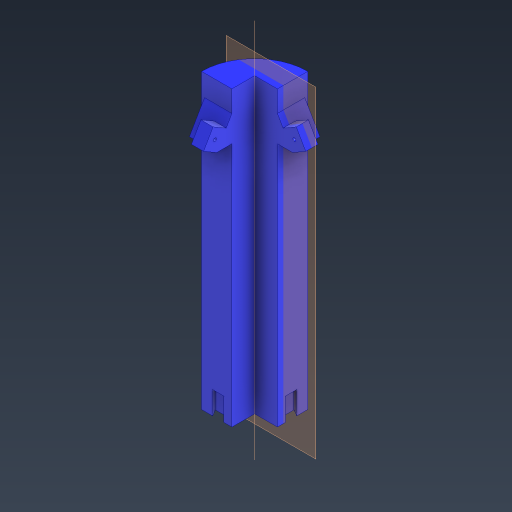
# Autodesk Inventor part: Край стен
Saved by Autodesk Inventor 2023.2 (Build 272271030, 271C)
## iProperties
Created: 2025-08-19
Part Number: Край стен
Material: Типовые
Document SubType Name: Modeling
Designer: Олег Коноваленко
Density: 1 g/cm^3
Appearance: Синий — малярная краска — глянцевая
Mass: 1127.71 g
Surface Area: 1041.8 cm^2
Volume: 1127.71 cm^3
Author: Олег Коноваленко
Autodesk Inventor part; units mm, degrees
ref_plane "YZ Plane" through (0, 0, 0) normal (1, 0, 0) x (0, 1, 0)
ref_plane "XZ Plane" through (0, 0, 0) normal (0, 1, 0) x (-1, 0, 0)
ref_plane "XY Plane" through (0, 0, 0) normal (0, 0, 1) x (1, 0, 0)
sketch "Эскиз1" plane through (0, 0, 0) normal (0, 1, 0) x (-1, 0, 0)
  line L0 (-39.7487, 9.7487) -> (-39.7487, -30.2513)
  line L1 (-9.7487, 9.7487) -> (-39.7487, 9.7487)
  line L2 (-9.7487, 9.7487) -> (-9.7487, 39.7487)
  line L3 (-9.7487, 39.7487) -> (30.2513, 39.7487)
  arc A0 (-39.7487, -30.2513) -> (30.2513, 39.7487) centre (-39.7487, 39.7487) ccw
  line L4 (-9.7487, 9.7487) -> (9.7487, -9.7487) construction
  point P0 (0, 0)
  point P1 (0, 0)
  dimension "d27" = 40
  dimension "d83" = 30
  constraints: 10 end point, 4 perpendicular, 3 point on circle, 2 line through centre, 1 centre point, 1 coincident, 1 horizontal, 1 midpoint, 1 vertical
  measures "d27" distance of L0.start L0.end
  measures "d83" distance of L1.start L0.start
extrude "Выдавливание16" add sketch "Эскиз1" along normal mid plane 386
ref_plane "РабПлоскость13" through (39.7487, 193, 39.7487) normal (-0.7071068, 0, 0.7071068) x (0, -1, 0)
sketch "Эскиз34" plane through (39.7487, 193, 39.7487) normal (-0.7071068, 0, 0.7071068) x (0, -1, 0)
  line L0 (-30, -100) -> (416, -100)
  line L1 (416, -100) -> (416, 8.7868)
  line L2 (416, 8.7868) -> (-30, 8.7868)
  line L3 (-30, 8.7868) -> (-30, -100)
  line L4 (386, -70) -> (0, -70) projected
  line L5 (386, -21.2132) -> (0, -21.2132) projected
  line L6 (386, -21.2132) -> (386, -49.4975) projected
  line L7 (0, -49.4975) -> (0, -21.2132) projected
  point P0 (193, -56.2132)
  dimension "d102" = 30
  dimension "d103" = 30
  dimension "d104" = 30
  dimension "d105" = 30
  constraints: 8 end point, 2 parallel, 1 horizontal, 1 perpendicular
  measures "d102" distance between parallel lines of L3 L7
  measures "d103" distance between parallel lines of L4 L0
  measures "d104" distance between parallel lines of L5 L2
  measures "d105" distance between parallel lines of L1 L6
sketch "Эскиз36" plane through (0, -193, 0) normal (0, -1, 0) x (1, 0, 0)
  line L0 (39.7487, 9.7487) -> (39.7487, -30.2513)
  line L1 (31.0885, -20.7513) -> (39.7487, -15.7513)
  line L2 (31.0885, 4.2487) -> (31.0885, -20.7513)
  line L3 (39.7487, -0.7513) -> (31.0885, 4.2487)
  point P0 (0, 0)
  constraints: 8 end point, 2 vertical, 8 other
extrude "Выдавливание25" cut sketch "Эскиз36" against normal blind 30
extrude "Выдавливание23" [suppressed]
mirror "Зеркальное отражение4" about plane through (39.7487, 193, 39.7487) normal (-0.7071068, 0, 0.7071068) of "Выдавливание25"
sketch "Эскиз37" plane through (9.7487, -193, 39.7487) normal (1, 0, 0) x (0, 0, -1)
  line L0 (-8.2128, 343.7788) -> (-180.7128, 45)
  line L1 (0, 0) -> (0, 386) projected
  line L2 (0, 358.0038) -> (-20, 323.3628)
  line L3 (-20, 323.3628) -> (0, 323.3628)
  point P0 (39.7487, 193)
  point P1 (-20, 323.3628)
  dimension "d112" = 30
  dimension "d113" = 20
  constraints: 6 end point, 3 point on line, 1 horizontal, 3 other
  measures "d112" angle of L1 L2
  measures "d113" distance of L2.end L3.end
ref_plane "РабПлоскость14" through (-26.2513, -147.25, 49.2606) normal (-1, 0, 0) x (0, 0.5, 0.8660254)
extrude "Выдавливание26" add sketch "Эскиз37" against normal up to surface (36 mm away)
sketch "Эскиз38" plane through (-26.2513, 130.3628, 59.7487) normal (0, 0.5, 0.8660254) x (1, 0, 0)
  line L0 (36, 0) -> (36, 10) projected
  line L1 (36, 0) -> (20, 0)
  line L2 (20, 0) -> (20, 25)
  line L3 (20, 25) -> (36, 25)
  line L4 (36, 25) -> (36, 0)
  point P0 (26.2513, -83.0231)
  dimension "d116" = 16
  dimension "d117" = 25
  constraints: 8 end point, 2 parallel, 1 horizontal, 1 perpendicular
  measures "d116" distance of L2.end L3.end
  measures "d117" distance of L3.end L0.start
extrude "Выдавливание27" add sketch "Эскиз38" along normal blind 20
sketch "Эскиз39" plane through (9.7487, -193, 9.7487) normal (1, 0, 0) x (0, 0, -1)
  circle A0 centre (-52.4103, 339.1881) radius 2.1
  point P0 (9.7487, 193)
  constraints: 1 centre point, 2 other
extrude "Выдавливание28" cut sketch "Эскиз39" against normal blind 10
extrude "Выдавливание24" [suppressed]
mirror "Зеркальное отражение5" about plane through (39.7487, 193, 39.7487) normal (-0.7071068, 0, 0.7071068) of "Выдавливание26", "Выдавливание27", "Выдавливание28"
ref_plane "РабПлоскость16" through (-6.2513, 141.1881, 53.4987) normal (0, -0.8660254, 0.5) x (1, 0, 0)
ref_plane "РабПлоскость17" through (9.7487, 193, 1.7487) normal (0, 0, 1) x (1, 0, 0)
ref_plane "РабПлоскость18" through (53.4987, 141.1881, -6.2513) normal (0.5, -0.8660254, 0) x (0.8660254, 0.5, 0)
